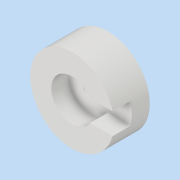
# Autodesk Inventor part: EncoderDisc
Saved by Autodesk Inventor 2017 (Build 210142000, 142)
## iProperties
Created: 2017-11-01
Part Number: EncoderDisc
Material: ABS Plastic
Document SubType Name: Modeling
Designer: Derek Wider
Density: 1.06 g/cm^3
Appearance: Smooth - White
Author: Derek Wider
Autodesk Inventor part; units mm, degrees
ref_plane "YZ Plane" through (0, 0, 0) normal (1, 0, 0) x (0, 1, 0)
ref_plane "XZ Plane" through (0, 0, 0) normal (0, 1, 0) x (-1, 0, 0)
ref_plane "XY Plane" through (0, 0, 0) normal (0, 0, 1) x (1, 0, 0)
sketch "Sketch1" plane through (0, 0, 0) normal (0, 0, 1) x (1, 0, 0)
  circle A0 centre (0, 0) radius 11.1125
  circle A1 centre (0, 0) radius 5.5245
  circle A2 centre (0, 0) radius 1.8415
  dimension "d0" = 22.225
  dimension "d1" = 11.049
  dimension "d2" = 3.683
  constraints: 3 centre point, 3 coincident
  measures "d0" diameter of A0
  measures "d1" diameter of A1
  measures "d2" diameter of A2
extrude "Extrusion1" add sketch "Sketch1" along normal blind 9.525 contours A0
extrude "Extrusion2" add sketch "Sketch1" along normal blind 4.7625 contours A1
sketch "Sketch2" plane through (0, 0, 0) normal (1, 0, 0) x (0, 1, 0)
  line L0 (11.1125, 9.525) -> (-11.1125, 9.525) projected
  line L1 (2.8575, 9.525) -> (-2.8575, 9.525)
  line L2 (-2.8575, 9.525) -> (-2.8575, 4.7625)
  line L3 (-2.8575, 4.7625) -> (2.8575, 4.7625)
  line L4 (2.8575, 4.7625) -> (2.8575, 9.525)
  point P0 (0, 0)
  dimension "d7" = 5.715
  dimension "d8" = 2.8575
  dimension "d9" = 4.7625
  constraints: 8 end point, 2 parallel, 1 horizontal, 1 perpendicular, 1 point on line
  measures "d7" distance between parallel lines of L2 L4
  measures "d8" distance from line of point (0, 0) L2
  measures "d9" distance of L3.end L1.start
extrude "Extrusion3" cut sketch "Sketch2" along normal through all
equation "\"d5\" = 0.5 * d3"
equation "\"d8\" = 0.5 * d7"
equation "\"d10\" = 0.5 * d3"
equation "\"d3\" = 9.525"
body "Solid1"
